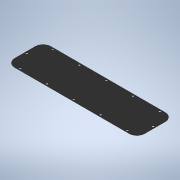
# Autodesk Inventor part: CAD_FPL_1060.000
Saved by Autodesk Inventor 2021 (Build 250183000, 183)
## iProperties
Created: 2025-09-22
Part Number: CAD_FPL_1060.000
Material: Generic
Catalog Web Link: www.cadenas.de
Description: Gland plate AX-Compact enclosures
Vendor: RITTAL
Document SubType Name: Modeling
Designer: psAdmin
Manufacturer: RITTAL
Mass: 117.298 g
Surface Area: 1587.71 cm^2
Volume: 117.298 cm^3
Density: 1 g/cm^3
Appearance: PSOLRGB-175-175-175
Category: PARTsolutions
Company: RITTAL
Title: CAD_FPL_1060.000
Author: Cadenas PARTsolutions
Comments: Compact enclosures
PSOL_IDENT_0: {$CADENAS_DATA/23d-libs/rittal/schaltschranksys/ausbauteile_cad/flanschplatten/ae_2_0_sep_fpl.prj},1
PSOL_IDENT_1: 81 {VTYP=3D},{NB=CAD_FPL_1060.000},{LINA=CAD_FPL_1060.000},{NN=Gland plate AX},{DATE=28.04.2025 21:1
PSOL_IDENT_2: 0:23},{GEOMDATE=11.04.2025 07:45:17},{VERSION=},{LINEID=350},{WBVAR=},{WBNUMERIC=}  {NB=CAD_FPL_1060
PSOL_IDENT_3: .000},{LINA=CAD_FPL_1060.000},{KT=DUMMY},{BEST=CAD_FPL_1060.000},{DETAIL=1},{VERS=7},{D=534},{E=149}
PSOL_IDENT_4: ,{BEZ1=Neues Kompaktgehäuse},{BEZ2=Stahlblech},{BEZ3=eintürig},{TUER=1},{B=600},{H=600},{T=210},{F=5
PSOL_IDENT_5: 50},{G=575},{B1=600},{B3=560.000},{B4=470.000},{B5=498.000},{BB5=0.000},{H1=600},{H3=560.000},{H4=85
PSOL_IDENT_6: .000},{H5=113.000},{HH5=4.000},{T5=93.500},{R1=31.000},{R2=8.000},{T1=210},{F1=550},{G1=575},{ST=MIN
PSOL_IDENT_7: },{VERS3=0},{CNSECLASS51=27-18-01-02},{CNSECLASS70=27-18-01-01},{CNSECLASS80=27-18-01-01},{CNSETIM40=
PSOL_IDENT_8: EC000261},{S=1.50},{W=600.000},{W1=556.000},{W2=500.000},{HH=600.000},{HH1=556.000},{HH2=550.000},{H
PSOL_IDENT_9: H3=475.000},{D1=205.100},{VERS1=1}
NB: CAD_FPL_1060.000
NN: Gland plate AX
NT: Compact enclosures
NBSYN: $BEST.
LINA: CAD_FPL_1060.000
CATALOG: Rittal
BEST: CAD_FPL_1060.000
D: 534
E: 149
SUPPLIER: RITTAL
ARTICLENO: CAD_FPL_1060.000
BOMINFO: CAD_FPL_1060.000
CREATOR: CADENAS GmbH
Autodesk Inventor part; units mm, degrees
(part 1 of 3)
sketch "Sketch_7" plane through (0, 0, 0) normal (0, 1, 0) x (1, 0, 0)
  arc A0 (-267, -42.5) -> (-235, -74.5) centre (-235, -42.5) ccw
  line L0 (-235, -74.5) -> (235, -74.5)
  arc A1 (235, -74.5) -> (267, -42.5) centre (235, -42.5) ccw
  line L1 (267, -42.5) -> (267, 42.5)
  arc A2 (267, 42.5) -> (235, 74.5) centre (235, 42.5) ccw
  line L2 (235, 74.5) -> (-235, 74.5)
  arc A3 (-235, 74.5) -> (-267, 42.5) centre (-235, 42.5) ccw
  line L3 (-267, 42.5) -> (-267, -42.5)
  circle A4 centre (259, 0) radius 3.6
  circle A5 centre (220, -66.5) radius 3.6
  circle A6 centre (220, 66.5) radius 3.6
  circle A7 centre (110, -66.5) radius 3.6
  circle A8 centre (110, 66.5) radius 3.6
  circle A9 centre (0, -66.5) radius 3.6
  circle A10 centre (0, 66.5) radius 3.6
  circle A11 centre (-110, -66.5) radius 3.6
  circle A12 centre (-110, 66.5) radius 3.6
  circle A13 centre (-220, -66.5) radius 3.6
  circle A14 centre (-220, 66.5) radius 3.6
  circle A15 centre (-259, 0) radius 3.6
  constraints: 16 centre point, 8 end point, 8 point on circle
extrude "Extrusion1" add sketch "Sketch_7" along normal blind 1.5
ref_plane "FP_XY" through (0, 0, 0) normal (0, -1, 0) x (1, 0, 0)
ref_plane "FP_YZ" through (0, 0, 0) normal (1, 0, 0) x (0, 0, 1)
ref_plane "FP_ZX" through (0, 0, 0) normal (0, 0, 1) x (0, -1, 0)
ref_plane "to_Bolt_1_XY" through (-300, 0, -300) normal (0, 1, 0) x (1, 0, 0)
ref_plane "to_Bolt_1_YZ" through (-300, 0, -300) normal (1, 0, 0) x (0, 0, -1)
ref_plane "to_Bolt_1_ZX" through (-300, 0, -300) normal (0, 0, -1) x (0, 1, 0)
ref_plane "to_Bolt_1_1_XY" through (-300, 0, -300) normal (0, 1, 0) x (1, 0, 0)
ref_plane "to_Bolt_1_1_YZ" through (-300, 0, -300) normal (1, 0, 0) x (0, 0, -1)
ref_plane "to_Bolt_1_1_ZX" through (-300, 0, -300) normal (0, 0, -1) x (0, 1, 0)
ref_plane "to_Bolt_1_10_XY" through (-274.1627, 0, -300) normal (0, 1, 0) x (1, 0, 0)
ref_plane "to_Bolt_1_10_YZ" through (-274.1627, 0, -300) normal (1, 0, 0) x (0, 0, -1)
ref_plane "to_Bolt_1_10_ZX" through (-274.1627, 0, -300) normal (0, 0, -1) x (0, 1, 0)
ref_plane "to_Bolt_1_100_XY" through (-15.7895, 0, -300) normal (0, 1, 0) x (1, 0, 0)
ref_plane "to_Bolt_1_100_YZ" through (-15.7895, 0, -300) normal (1, 0, 0) x (0, 0, -1)
ref_plane "to_Bolt_1_100_ZX" through (-15.7895, 0, -300) normal (0, 0, -1) x (0, 1, 0)
ref_plane "to_Bolt_1_101_XY" through (-12.9187, 0, -300) normal (0, 1, 0) x (1, 0, 0)
ref_plane "to_Bolt_1_101_YZ" through (-12.9187, 0, -300) normal (1, 0, 0) x (0, 0, -1)
ref_plane "to_Bolt_1_101_ZX" through (-12.9187, 0, -300) normal (0, 0, -1) x (0, 1, 0)
ref_plane "to_Bolt_1_102_XY" through (-10.0478, 0, -300) normal (0, 1, 0) x (1, 0, 0)
ref_plane "to_Bolt_1_102_YZ" through (-10.0478, 0, -300) normal (1, 0, 0) x (0, 0, -1)
ref_plane "to_Bolt_1_102_ZX" through (-10.0478, 0, -300) normal (0, 0, -1) x (0, 1, 0)
ref_plane "to_Bolt_1_103_XY" through (-7.177, 0, -300) normal (0, 1, 0) x (1, 0, 0)
ref_plane "to_Bolt_1_103_YZ" through (-7.177, 0, -300) normal (1, 0, 0) x (0, 0, -1)
ref_plane "to_Bolt_1_103_ZX" through (-7.177, 0, -300) normal (0, 0, -1) x (0, 1, 0)
ref_plane "to_Bolt_1_104_XY" through (-4.3062, 0, -300) normal (0, 1, 0) x (1, 0, 0)
ref_plane "to_Bolt_1_104_YZ" through (-4.3062, 0, -300) normal (1, 0, 0) x (0, 0, -1)
ref_plane "to_Bolt_1_104_ZX" through (-4.3062, 0, -300) normal (0, 0, -1) x (0, 1, 0)
ref_plane "to_Bolt_1_105_XY" through (-1.4354, 0, -300) normal (0, 1, 0) x (1, 0, 0)
ref_plane "to_Bolt_1_105_YZ" through (-1.4354, 0, -300) normal (1, 0, 0) x (0, 0, -1)
ref_plane "to_Bolt_1_105_ZX" through (-1.4354, 0, -300) normal (0, 0, -1) x (0, 1, 0)
ref_plane "to_Bolt_1_106_XY" through (1.4354, 0, -300) normal (0, 1, 0) x (1, 0, 0)
ref_plane "to_Bolt_1_106_YZ" through (1.4354, 0, -300) normal (1, 0, 0) x (0, 0, -1)
ref_plane "to_Bolt_1_106_ZX" through (1.4354, 0, -300) normal (0, 0, -1) x (0, 1, 0)
ref_plane "to_Bolt_1_107_XY" through (4.3062, 0, -300) normal (0, 1, 0) x (1, 0, 0)
ref_plane "to_Bolt_1_107_YZ" through (4.3062, 0, -300) normal (1, 0, 0) x (0, 0, -1)
ref_plane "to_Bolt_1_107_ZX" through (4.3062, 0, -300) normal (0, 0, -1) x (0, 1, 0)
ref_plane "to_Bolt_1_108_XY" through (7.177, 0, -300) normal (0, 1, 0) x (1, 0, 0)
ref_plane "to_Bolt_1_108_YZ" through (7.177, 0, -300) normal (1, 0, 0) x (0, 0, -1)
ref_plane "to_Bolt_1_108_ZX" through (7.177, 0, -300) normal (0, 0, -1) x (0, 1, 0)
ref_plane "to_Bolt_1_109_XY" through (10.0478, 0, -300) normal (0, 1, 0) x (1, 0, 0)
ref_plane "to_Bolt_1_109_YZ" through (10.0478, 0, -300) normal (1, 0, 0) x (0, 0, -1)
ref_plane "to_Bolt_1_109_ZX" through (10.0478, 0, -300) normal (0, 0, -1) x (0, 1, 0)
ref_plane "to_Bolt_1_11_XY" through (-271.2919, 0, -300) normal (0, 1, 0) x (1, 0, 0)
ref_plane "to_Bolt_1_11_YZ" through (-271.2919, 0, -300) normal (1, 0, 0) x (0, 0, -1)
ref_plane "to_Bolt_1_11_ZX" through (-271.2919, 0, -300) normal (0, 0, -1) x (0, 1, 0)
ref_plane "to_Bolt_1_110_XY" through (12.9187, 0, -300) normal (0, 1, 0) x (1, 0, 0)
ref_plane "to_Bolt_1_110_YZ" through (12.9187, 0, -300) normal (1, 0, 0) x (0, 0, -1)
ref_plane "to_Bolt_1_110_ZX" through (12.9187, 0, -300) normal (0, 0, -1) x (0, 1, 0)
ref_plane "to_Bolt_1_111_XY" through (15.7895, 0, -300) normal (0, 1, 0) x (1, 0, 0)
ref_plane "to_Bolt_1_111_YZ" through (15.7895, 0, -300) normal (1, 0, 0) x (0, 0, -1)
ref_plane "to_Bolt_1_111_ZX" through (15.7895, 0, -300) normal (0, 0, -1) x (0, 1, 0)
ref_plane "to_Bolt_1_112_XY" through (18.6603, 0, -300) normal (0, 1, 0) x (1, 0, 0)
ref_plane "to_Bolt_1_112_YZ" through (18.6603, 0, -300) normal (1, 0, 0) x (0, 0, -1)
ref_plane "to_Bolt_1_112_ZX" through (18.6603, 0, -300) normal (0, 0, -1) x (0, 1, 0)
ref_plane "to_Bolt_1_113_XY" through (21.5311, 0, -300) normal (0, 1, 0) x (1, 0, 0)
ref_plane "to_Bolt_1_113_YZ" through (21.5311, 0, -300) normal (1, 0, 0) x (0, 0, -1)
ref_plane "to_Bolt_1_113_ZX" through (21.5311, 0, -300) normal (0, 0, -1) x (0, 1, 0)
ref_plane "to_Bolt_1_114_XY" through (24.4019, 0, -300) normal (0, 1, 0) x (1, 0, 0)
ref_plane "to_Bolt_1_114_YZ" through (24.4019, 0, -300) normal (1, 0, 0) x (0, 0, -1)
ref_plane "to_Bolt_1_114_ZX" through (24.4019, 0, -300) normal (0, 0, -1) x (0, 1, 0)
ref_plane "to_Bolt_1_115_XY" through (27.2727, 0, -300) normal (0, 1, 0) x (1, 0, 0)
ref_plane "to_Bolt_1_115_YZ" through (27.2727, 0, -300) normal (1, 0, 0) x (0, 0, -1)
ref_plane "to_Bolt_1_115_ZX" through (27.2727, 0, -300) normal (0, 0, -1) x (0, 1, 0)
ref_plane "to_Bolt_1_116_XY" through (30.1435, 0, -300) normal (0, 1, 0) x (1, 0, 0)
ref_plane "to_Bolt_1_116_YZ" through (30.1435, 0, -300) normal (1, 0, 0) x (0, 0, -1)
ref_plane "to_Bolt_1_116_ZX" through (30.1435, 0, -300) normal (0, 0, -1) x (0, 1, 0)
ref_plane "to_Bolt_1_117_XY" through (33.0144, 0, -300) normal (0, 1, 0) x (1, 0, 0)
ref_plane "to_Bolt_1_117_YZ" through (33.0144, 0, -300) normal (1, 0, 0) x (0, 0, -1)
ref_plane "to_Bolt_1_117_ZX" through (33.0144, 0, -300) normal (0, 0, -1) x (0, 1, 0)
ref_plane "to_Bolt_1_118_XY" through (35.8852, 0, -300) normal (0, 1, 0) x (1, 0, 0)
ref_plane "to_Bolt_1_118_YZ" through (35.8852, 0, -300) normal (1, 0, 0) x (0, 0, -1)
ref_plane "to_Bolt_1_118_ZX" through (35.8852, 0, -300) normal (0, 0, -1) x (0, 1, 0)
ref_plane "to_Bolt_1_119_XY" through (38.756, 0, -300) normal (0, 1, 0) x (1, 0, 0)
ref_plane "to_Bolt_1_119_YZ" through (38.756, 0, -300) normal (1, 0, 0) x (0, 0, -1)
ref_plane "to_Bolt_1_119_ZX" through (38.756, 0, -300) normal (0, 0, -1) x (0, 1, 0)
ref_plane "to_Bolt_1_12_XY" through (-268.4211, 0, -300) normal (0, 1, 0) x (1, 0, 0)
ref_plane "to_Bolt_1_12_YZ" through (-268.4211, 0, -300) normal (1, 0, 0) x (0, 0, -1)
ref_plane "to_Bolt_1_12_ZX" through (-268.4211, 0, -300) normal (0, 0, -1) x (0, 1, 0)
ref_plane "to_Bolt_1_120_XY" through (41.6268, 0, -300) normal (0, 1, 0) x (1, 0, 0)
ref_plane "to_Bolt_1_120_YZ" through (41.6268, 0, -300) normal (1, 0, 0) x (0, 0, -1)
ref_plane "to_Bolt_1_120_ZX" through (41.6268, 0, -300) normal (0, 0, -1) x (0, 1, 0)
ref_plane "to_Bolt_1_121_XY" through (44.4976, 0, -300) normal (0, 1, 0) x (1, 0, 0)
ref_plane "to_Bolt_1_121_YZ" through (44.4976, 0, -300) normal (1, 0, 0) x (0, 0, -1)
ref_plane "to_Bolt_1_121_ZX" through (44.4976, 0, -300) normal (0, 0, -1) x (0, 1, 0)
ref_plane "to_Bolt_1_122_XY" through (47.3684, 0, -300) normal (0, 1, 0) x (1, 0, 0)
ref_plane "to_Bolt_1_122_YZ" through (47.3684, 0, -300) normal (1, 0, 0) x (0, 0, -1)
ref_plane "to_Bolt_1_122_ZX" through (47.3684, 0, -300) normal (0, 0, -1) x (0, 1, 0)
ref_plane "to_Bolt_1_123_XY" through (50.2392, 0, -300) normal (0, 1, 0) x (1, 0, 0)
ref_plane "to_Bolt_1_123_YZ" through (50.2392, 0, -300) normal (1, 0, 0) x (0, 0, -1)
ref_plane "to_Bolt_1_123_ZX" through (50.2392, 0, -300) normal (0, 0, -1) x (0, 1, 0)
ref_plane "to_Bolt_1_124_XY" through (53.11, 0, -300) normal (0, 1, 0) x (1, 0, 0)
ref_plane "to_Bolt_1_124_YZ" through (53.11, 0, -300) normal (1, 0, 0) x (0, 0, -1)
ref_plane "to_Bolt_1_124_ZX" through (53.11, 0, -300) normal (0, 0, -1) x (0, 1, 0)
ref_plane "to_Bolt_1_125_XY" through (55.9809, 0, -300) normal (0, 1, 0) x (1, 0, 0)
ref_plane "to_Bolt_1_125_YZ" through (55.9809, 0, -300) normal (1, 0, 0) x (0, 0, -1)
ref_plane "to_Bolt_1_125_ZX" through (55.9809, 0, -300) normal (0, 0, -1) x (0, 1, 0)
ref_plane "to_Bolt_1_126_XY" through (58.8517, 0, -300) normal (0, 1, 0) x (1, 0, 0)
ref_plane "to_Bolt_1_126_YZ" through (58.8517, 0, -300) normal (1, 0, 0) x (0, 0, -1)
ref_plane "to_Bolt_1_126_ZX" through (58.8517, 0, -300) normal (0, 0, -1) x (0, 1, 0)
ref_plane "to_Bolt_1_127_XY" through (61.7225, 0, -300) normal (0, 1, 0) x (1, 0, 0)
ref_plane "to_Bolt_1_127_YZ" through (61.7225, 0, -300) normal (1, 0, 0) x (0, 0, -1)
ref_plane "to_Bolt_1_127_ZX" through (61.7225, 0, -300) normal (0, 0, -1) x (0, 1, 0)
ref_plane "to_Bolt_1_128_XY" through (64.5933, 0, -300) normal (0, 1, 0) x (1, 0, 0)
ref_plane "to_Bolt_1_128_YZ" through (64.5933, 0, -300) normal (1, 0, 0) x (0, 0, -1)
ref_plane "to_Bolt_1_128_ZX" through (64.5933, 0, -300) normal (0, 0, -1) x (0, 1, 0)
ref_plane "to_Bolt_1_129_XY" through (67.4641, 0, -300) normal (0, 1, 0) x (1, 0, 0)
ref_plane "to_Bolt_1_129_YZ" through (67.4641, 0, -300) normal (1, 0, 0) x (0, 0, -1)
ref_plane "to_Bolt_1_129_ZX" through (67.4641, 0, -300) normal (0, 0, -1) x (0, 1, 0)
ref_plane "to_Bolt_1_13_XY" through (-265.5502, 0, -300) normal (0, 1, 0) x (1, 0, 0)
ref_plane "to_Bolt_1_13_YZ" through (-265.5502, 0, -300) normal (1, 0, 0) x (0, 0, -1)
ref_plane "to_Bolt_1_13_ZX" through (-265.5502, 0, -300) normal (0, 0, -1) x (0, 1, 0)
ref_plane "to_Bolt_1_130_XY" through (70.3349, 0, -300) normal (0, 1, 0) x (1, 0, 0)
ref_plane "to_Bolt_1_130_YZ" through (70.3349, 0, -300) normal (1, 0, 0) x (0, 0, -1)
ref_plane "to_Bolt_1_130_ZX" through (70.3349, 0, -300) normal (0, 0, -1) x (0, 1, 0)
ref_plane "to_Bolt_1_131_XY" through (73.2057, 0, -300) normal (0, 1, 0) x (1, 0, 0)
ref_plane "to_Bolt_1_131_YZ" through (73.2057, 0, -300) normal (1, 0, 0) x (0, 0, -1)
ref_plane "to_Bolt_1_131_ZX" through (73.2057, 0, -300) normal (0, 0, -1) x (0, 1, 0)
ref_plane "to_Bolt_1_132_XY" through (76.0766, 0, -300) normal (0, 1, 0) x (1, 0, 0)
ref_plane "to_Bolt_1_132_YZ" through (76.0766, 0, -300) normal (1, 0, 0) x (0, 0, -1)
ref_plane "to_Bolt_1_132_ZX" through (76.0766, 0, -300) normal (0, 0, -1) x (0, 1, 0)
ref_plane "to_Bolt_1_133_XY" through (78.9474, 0, -300) normal (0, 1, 0) x (1, 0, 0)
ref_plane "to_Bolt_1_133_YZ" through (78.9474, 0, -300) normal (1, 0, 0) x (0, 0, -1)
ref_plane "to_Bolt_1_133_ZX" through (78.9474, 0, -300) normal (0, 0, -1) x (0, 1, 0)
ref_plane "to_Bolt_1_134_XY" through (81.8182, 0, -300) normal (0, 1, 0) x (1, 0, 0)
ref_plane "to_Bolt_1_134_YZ" through (81.8182, 0, -300) normal (1, 0, 0) x (0, 0, -1)
ref_plane "to_Bolt_1_134_ZX" through (81.8182, 0, -300) normal (0, 0, -1) x (0, 1, 0)
ref_plane "to_Bolt_1_135_XY" through (84.689, 0, -300) normal (0, 1, 0) x (1, 0, 0)
ref_plane "to_Bolt_1_135_YZ" through (84.689, 0, -300) normal (1, 0, 0) x (0, 0, -1)
ref_plane "to_Bolt_1_135_ZX" through (84.689, 0, -300) normal (0, 0, -1) x (0, 1, 0)
ref_plane "to_Bolt_1_136_XY" through (87.5598, 0, -300) normal (0, 1, 0) x (1, 0, 0)
ref_plane "to_Bolt_1_136_YZ" through (87.5598, 0, -300) normal (1, 0, 0) x (0, 0, -1)
ref_plane "to_Bolt_1_136_ZX" through (87.5598, 0, -300) normal (0, 0, -1) x (0, 1, 0)
ref_plane "to_Bolt_1_137_XY" through (90.4306, 0, -300) normal (0, 1, 0) x (1, 0, 0)
ref_plane "to_Bolt_1_137_YZ" through (90.4306, 0, -300) normal (1, 0, 0) x (0, 0, -1)
ref_plane "to_Bolt_1_137_ZX" through (90.4306, 0, -300) normal (0, 0, -1) x (0, 1, 0)
ref_plane "to_Bolt_1_138_XY" through (93.3014, 0, -300) normal (0, 1, 0) x (1, 0, 0)
ref_plane "to_Bolt_1_138_YZ" through (93.3014, 0, -300) normal (1, 0, 0) x (0, 0, -1)
ref_plane "to_Bolt_1_138_ZX" through (93.3014, 0, -300) normal (0, 0, -1) x (0, 1, 0)
ref_plane "to_Bolt_1_139_XY" through (96.1722, 0, -300) normal (0, 1, 0) x (1, 0, 0)
ref_plane "to_Bolt_1_139_YZ" through (96.1722, 0, -300) normal (1, 0, 0) x (0, 0, -1)
ref_plane "to_Bolt_1_139_ZX" through (96.1722, 0, -300) normal (0, 0, -1) x (0, 1, 0)
ref_plane "to_Bolt_1_14_XY" through (-262.6794, 0, -300) normal (0, 1, 0) x (1, 0, 0)
ref_plane "to_Bolt_1_14_YZ" through (-262.6794, 0, -300) normal (1, 0, 0) x (0, 0, -1)
ref_plane "to_Bolt_1_14_ZX" through (-262.6794, 0, -300) normal (0, 0, -1) x (0, 1, 0)
ref_plane "to_Bolt_1_140_XY" through (99.0431, 0, -300) normal (0, 1, 0) x (1, 0, 0)
ref_plane "to_Bolt_1_140_YZ" through (99.0431, 0, -300) normal (1, 0, 0) x (0, 0, -1)
ref_plane "to_Bolt_1_140_ZX" through (99.0431, 0, -300) normal (0, 0, -1) x (0, 1, 0)
ref_plane "to_Bolt_1_141_XY" through (101.9139, 0, -300) normal (0, 1, 0) x (1, 0, 0)
ref_plane "to_Bolt_1_141_YZ" through (101.9139, 0, -300) normal (1, 0, 0) x (0, 0, -1)
ref_plane "to_Bolt_1_141_ZX" through (101.9139, 0, -300) normal (0, 0, -1) x (0, 1, 0)
ref_plane "to_Bolt_1_142_XY" through (104.7847, 0, -300) normal (0, 1, 0) x (1, 0, 0)
ref_plane "to_Bolt_1_142_YZ" through (104.7847, 0, -300) normal (1, 0, 0) x (0, 0, -1)
ref_plane "to_Bolt_1_142_ZX" through (104.7847, 0, -300) normal (0, 0, -1) x (0, 1, 0)
ref_plane "to_Bolt_1_143_XY" through (107.6555, 0, -300) normal (0, 1, 0) x (1, 0, 0)
ref_plane "to_Bolt_1_143_YZ" through (107.6555, 0, -300) normal (1, 0, 0) x (0, 0, -1)
ref_plane "to_Bolt_1_143_ZX" through (107.6555, 0, -300) normal (0, 0, -1) x (0, 1, 0)
ref_plane "to_Bolt_1_144_XY" through (110.5263, 0, -300) normal (0, 1, 0) x (1, 0, 0)
ref_plane "to_Bolt_1_144_YZ" through (110.5263, 0, -300) normal (1, 0, 0) x (0, 0, -1)
ref_plane "to_Bolt_1_144_ZX" through (110.5263, 0, -300) normal (0, 0, -1) x (0, 1, 0)
ref_plane "to_Bolt_1_145_XY" through (113.3971, 0, -300) normal (0, 1, 0) x (1, 0, 0)
ref_plane "to_Bolt_1_145_YZ" through (113.3971, 0, -300) normal (1, 0, 0) x (0, 0, -1)
ref_plane "to_Bolt_1_145_ZX" through (113.3971, 0, -300) normal (0, 0, -1) x (0, 1, 0)
ref_plane "to_Bolt_1_146_XY" through (116.2679, 0, -300) normal (0, 1, 0) x (1, 0, 0)
ref_plane "to_Bolt_1_146_YZ" through (116.2679, 0, -300) normal (1, 0, 0) x (0, 0, -1)
ref_plane "to_Bolt_1_146_ZX" through (116.2679, 0, -300) normal (0, 0, -1) x (0, 1, 0)
ref_plane "to_Bolt_1_147_XY" through (119.1388, 0, -300) normal (0, 1, 0) x (1, 0, 0)
ref_plane "to_Bolt_1_147_YZ" through (119.1388, 0, -300) normal (1, 0, 0) x (0, 0, -1)
ref_plane "to_Bolt_1_147_ZX" through (119.1388, 0, -300) normal (0, 0, -1) x (0, 1, 0)
ref_plane "to_Bolt_1_148_XY" through (122.0096, 0, -300) normal (0, 1, 0) x (1, 0, 0)
ref_plane "to_Bolt_1_148_YZ" through (122.0096, 0, -300) normal (1, 0, 0) x (0, 0, -1)
ref_plane "to_Bolt_1_148_ZX" through (122.0096, 0, -300) normal (0, 0, -1) x (0, 1, 0)
ref_plane "to_Bolt_1_149_XY" through (124.8804, 0, -300) normal (0, 1, 0) x (1, 0, 0)
ref_plane "to_Bolt_1_149_YZ" through (124.8804, 0, -300) normal (1, 0, 0) x (0, 0, -1)
ref_plane "to_Bolt_1_149_ZX" through (124.8804, 0, -300) normal (0, 0, -1) x (0, 1, 0)
ref_plane "to_Bolt_1_15_XY" through (-259.8086, 0, -300) normal (0, 1, 0) x (1, 0, 0)
ref_plane "to_Bolt_1_15_YZ" through (-259.8086, 0, -300) normal (1, 0, 0) x (0, 0, -1)
ref_plane "to_Bolt_1_15_ZX" through (-259.8086, 0, -300) normal (0, 0, -1) x (0, 1, 0)
ref_plane "to_Bolt_1_150_XY" through (127.7512, 0, -300) normal (0, 1, 0) x (1, 0, 0)
ref_plane "to_Bolt_1_150_YZ" through (127.7512, 0, -300) normal (1, 0, 0) x (0, 0, -1)
ref_plane "to_Bolt_1_150_ZX" through (127.7512, 0, -300) normal (0, 0, -1) x (0, 1, 0)
ref_plane "to_Bolt_1_151_XY" through (130.622, 0, -300) normal (0, 1, 0) x (1, 0, 0)
ref_plane "to_Bolt_1_151_YZ" through (130.622, 0, -300) normal (1, 0, 0) x (0, 0, -1)
ref_plane "to_Bolt_1_151_ZX" through (130.622, 0, -300) normal (0, 0, -1) x (0, 1, 0)
ref_plane "to_Bolt_1_152_XY" through (133.4928, 0, -300) normal (0, 1, 0) x (1, 0, 0)
ref_plane "to_Bolt_1_152_YZ" through (133.4928, 0, -300) normal (1, 0, 0) x (0, 0, -1)
ref_plane "to_Bolt_1_152_ZX" through (133.4928, 0, -300) normal (0, 0, -1) x (0, 1, 0)
ref_plane "to_Bolt_1_153_XY" through (136.3636, 0, -300) normal (0, 1, 0) x (1, 0, 0)
ref_plane "to_Bolt_1_153_YZ" through (136.3636, 0, -300) normal (1, 0, 0) x (0, 0, -1)
ref_plane "to_Bolt_1_153_ZX" through (136.3636, 0, -300) normal (0, 0, -1) x (0, 1, 0)
ref_plane "to_Bolt_1_154_XY" through (139.2344, 0, -300) normal (0, 1, 0) x (1, 0, 0)
ref_plane "to_Bolt_1_154_YZ" through (139.2344, 0, -300) normal (1, 0, 0) x (0, 0, -1)
ref_plane "to_Bolt_1_154_ZX" through (139.2344, 0, -300) normal (0, 0, -1) x (0, 1, 0)
ref_plane "to_Bolt_1_155_XY" through (142.1053, 0, -300) normal (0, 1, 0) x (1, 0, 0)
ref_plane "to_Bolt_1_155_YZ" through (142.1053, 0, -300) normal (1, 0, 0) x (0, 0, -1)
ref_plane "to_Bolt_1_155_ZX" through (142.1053, 0, -300) normal (0, 0, -1) x (0, 1, 0)
ref_plane "to_Bolt_1_156_XY" through (144.9761, 0, -300) normal (0, 1, 0) x (1, 0, 0)
ref_plane "to_Bolt_1_156_YZ" through (144.9761, 0, -300) normal (1, 0, 0) x (0, 0, -1)
ref_plane "to_Bolt_1_156_ZX" through (144.9761, 0, -300) normal (0, 0, -1) x (0, 1, 0)
ref_plane "to_Bolt_1_157_XY" through (147.8469, 0, -300) normal (0, 1, 0) x (1, 0, 0)
ref_plane "to_Bolt_1_157_YZ" through (147.8469, 0, -300) normal (1, 0, 0) x (0, 0, -1)
ref_plane "to_Bolt_1_157_ZX" through (147.8469, 0, -300) normal (0, 0, -1) x (0, 1, 0)
ref_plane "to_Bolt_1_158_XY" through (150.7177, 0, -300) normal (0, 1, 0) x (1, 0, 0)
ref_plane "to_Bolt_1_158_YZ" through (150.7177, 0, -300) normal (1, 0, 0) x (0, 0, -1)
ref_plane "to_Bolt_1_158_ZX" through (150.7177, 0, -300) normal (0, 0, -1) x (0, 1, 0)
ref_plane "to_Bolt_1_159_XY" through (153.5885, 0, -300) normal (0, 1, 0) x (1, 0, 0)
ref_plane "to_Bolt_1_159_YZ" through (153.5885, 0, -300) normal (1, 0, 0) x (0, 0, -1)
ref_plane "to_Bolt_1_159_ZX" through (153.5885, 0, -300) normal (0, 0, -1) x (0, 1, 0)
ref_plane "to_Bolt_1_16_XY" through (-256.9378, 0, -300) normal (0, 1, 0) x (1, 0, 0)
ref_plane "to_Bolt_1_16_YZ" through (-256.9378, 0, -300) normal (1, 0, 0) x (0, 0, -1)
ref_plane "to_Bolt_1_16_ZX" through (-256.9378, 0, -300) normal (0, 0, -1) x (0, 1, 0)
ref_plane "to_Bolt_1_160_XY" through (156.4593, 0, -300) normal (0, 1, 0) x (1, 0, 0)
ref_plane "to_Bolt_1_160_YZ" through (156.4593, 0, -300) normal (1, 0, 0) x (0, 0, -1)
ref_plane "to_Bolt_1_160_ZX" through (156.4593, 0, -300) normal (0, 0, -1) x (0, 1, 0)
ref_plane "to_Bolt_1_161_XY" through (159.3301, 0, -300) normal (0, 1, 0) x (1, 0, 0)
ref_plane "to_Bolt_1_161_YZ" through (159.3301, 0, -300) normal (1, 0, 0) x (0, 0, -1)
ref_plane "to_Bolt_1_161_ZX" through (159.3301, 0, -300) normal (0, 0, -1) x (0, 1, 0)
ref_plane "to_Bolt_1_162_XY" through (162.201, 0, -300) normal (0, 1, 0) x (1, 0, 0)
ref_plane "to_Bolt_1_162_YZ" through (162.201, 0, -300) normal (1, 0, 0) x (0, 0, -1)
ref_plane "to_Bolt_1_162_ZX" through (162.201, 0, -300) normal (0, 0, -1) x (0, 1, 0)
ref_plane "to_Bolt_1_163_XY" through (165.0718, 0, -300) normal (0, 1, 0) x (1, 0, 0)
ref_plane "to_Bolt_1_163_YZ" through (165.0718, 0, -300) normal (1, 0, 0) x (0, 0, -1)
ref_plane "to_Bolt_1_163_ZX" through (165.0718, 0, -300) normal (0, 0, -1) x (0, 1, 0)
ref_plane "to_Bolt_1_164_XY" through (167.9426, 0, -300) normal (0, 1, 0) x (1, 0, 0)
ref_plane "to_Bolt_1_164_YZ" through (167.9426, 0, -300) normal (1, 0, 0) x (0, 0, -1)
ref_plane "to_Bolt_1_164_ZX" through (167.9426, 0, -300) normal (0, 0, -1) x (0, 1, 0)
ref_plane "to_Bolt_1_165_XY" through (170.8134, 0, -300) normal (0, 1, 0) x (1, 0, 0)
ref_plane "to_Bolt_1_165_YZ" through (170.8134, 0, -300) normal (1, 0, 0) x (0, 0, -1)
ref_plane "to_Bolt_1_165_ZX" through (170.8134, 0, -300) normal (0, 0, -1) x (0, 1, 0)
ref_plane "to_Bolt_1_166_XY" through (173.6842, 0, -300) normal (0, 1, 0) x (1, 0, 0)
ref_plane "to_Bolt_1_166_YZ" through (173.6842, 0, -300) normal (1, 0, 0) x (0, 0, -1)
ref_plane "to_Bolt_1_166_ZX" through (173.6842, 0, -300) normal (0, 0, -1) x (0, 1, 0)
ref_plane "to_Bolt_1_167_XY" through (176.555, 0, -300) normal (0, 1, 0) x (1, 0, 0)
ref_plane "to_Bolt_1_167_YZ" through (176.555, 0, -300) normal (1, 0, 0) x (0, 0, -1)
ref_plane "to_Bolt_1_167_ZX" through (176.555, 0, -300) normal (0, 0, -1) x (0, 1, 0)
ref_plane "to_Bolt_1_168_XY" through (179.4258, 0, -300) normal (0, 1, 0) x (1, 0, 0)
ref_plane "to_Bolt_1_168_YZ" through (179.4258, 0, -300) normal (1, 0, 0) x (0, 0, -1)
ref_plane "to_Bolt_1_168_ZX" through (179.4258, 0, -300) normal (0, 0, -1) x (0, 1, 0)
ref_plane "to_Bolt_1_169_XY" through (182.2967, 0, -300) normal (0, 1, 0) x (1, 0, 0)
ref_plane "to_Bolt_1_169_YZ" through (182.2967, 0, -300) normal (1, 0, 0) x (0, 0, -1)
ref_plane "to_Bolt_1_169_ZX" through (182.2967, 0, -300) normal (0, 0, -1) x (0, 1, 0)
ref_plane "to_Bolt_1_17_XY" through (-254.067, 0, -300) normal (0, 1, 0) x (1, 0, 0)
ref_plane "to_Bolt_1_17_YZ" through (-254.067, 0, -300) normal (1, 0, 0) x (0, 0, -1)
ref_plane "to_Bolt_1_17_ZX" through (-254.067, 0, -300) normal (0, 0, -1) x (0, 1, 0)
ref_plane "to_Bolt_1_170_XY" through (185.1675, 0, -300) normal (0, 1, 0) x (1, 0, 0)
ref_plane "to_Bolt_1_170_YZ" through (185.1675, 0, -300) normal (1, 0, 0) x (0, 0, -1)
ref_plane "to_Bolt_1_170_ZX" through (185.1675, 0, -300) normal (0, 0, -1) x (0, 1, 0)
ref_plane "to_Bolt_1_171_XY" through (188.0383, 0, -300) normal (0, 1, 0) x (1, 0, 0)
ref_plane "to_Bolt_1_171_YZ" through (188.0383, 0, -300) normal (1, 0, 0) x (0, 0, -1)
ref_plane "to_Bolt_1_171_ZX" through (188.0383, 0, -300) normal (0, 0, -1) x (0, 1, 0)
ref_plane "to_Bolt_1_172_XY" through (190.9091, 0, -300) normal (0, 1, 0) x (1, 0, 0)
ref_plane "to_Bolt_1_172_YZ" through (190.9091, 0, -300) normal (1, 0, 0) x (0, 0, -1)
ref_plane "to_Bolt_1_172_ZX" through (190.9091, 0, -300) normal (0, 0, -1) x (0, 1, 0)
ref_plane "to_Bolt_1_173_XY" through (193.7799, 0, -300) normal (0, 1, 0) x (1, 0, 0)
ref_plane "to_Bolt_1_173_YZ" through (193.7799, 0, -300) normal (1, 0, 0) x (0, 0, -1)
ref_plane "to_Bolt_1_173_ZX" through (193.7799, 0, -300) normal (0, 0, -1) x (0, 1, 0)
ref_plane "to_Bolt_1_174_XY" through (196.6507, 0, -300) normal (0, 1, 0) x (1, 0, 0)
ref_plane "to_Bolt_1_174_YZ" through (196.6507, 0, -300) normal (1, 0, 0) x (0, 0, -1)
ref_plane "to_Bolt_1_174_ZX" through (196.6507, 0, -300) normal (0, 0, -1) x (0, 1, 0)
ref_plane "to_Bolt_1_175_XY" through (199.5215, 0, -300) normal (0, 1, 0) x (1, 0, 0)
ref_plane "to_Bolt_1_175_YZ" through (199.5215, 0, -300) normal (1, 0, 0) x (0, 0, -1)
ref_plane "to_Bolt_1_175_ZX" through (199.5215, 0, -300) normal (0, 0, -1) x (0, 1, 0)
ref_plane "to_Bolt_1_176_XY" through (202.3923, 0, -300) normal (0, 1, 0) x (1, 0, 0)
ref_plane "to_Bolt_1_176_YZ" through (202.3923, 0, -300) normal (1, 0, 0) x (0, 0, -1)
ref_plane "to_Bolt_1_176_ZX" through (202.3923, 0, -300) normal (0, 0, -1) x (0, 1, 0)
ref_plane "to_Bolt_1_177_XY" through (205.2632, 0, -300) normal (0, 1, 0) x (1, 0, 0)
ref_plane "to_Bolt_1_177_YZ" through (205.2632, 0, -300) normal (1, 0, 0) x (0, 0, -1)
ref_plane "to_Bolt_1_177_ZX" through (205.2632, 0, -300) normal (0, 0, -1) x (0, 1, 0)
ref_plane "to_Bolt_1_178_XY" through (208.134, 0, -300) normal (0, 1, 0) x (1, 0, 0)
ref_plane "to_Bolt_1_178_YZ" through (208.134, 0, -300) normal (1, 0, 0) x (0, 0, -1)
ref_plane "to_Bolt_1_178_ZX" through (208.134, 0, -300) normal (0, 0, -1) x (0, 1, 0)
ref_plane "to_Bolt_1_179_XY" through (211.0048, 0, -300) normal (0, 1, 0) x (1, 0, 0)
ref_plane "to_Bolt_1_179_YZ" through (211.0048, 0, -300) normal (1, 0, 0) x (0, 0, -1)
ref_plane "to_Bolt_1_179_ZX" through (211.0048, 0, -300) normal (0, 0, -1) x (0, 1, 0)
ref_plane "to_Bolt_1_18_XY" through (-251.1962, 0, -300) normal (0, 1, 0) x (1, 0, 0)
ref_plane "to_Bolt_1_18_YZ" through (-251.1962, 0, -300) normal (1, 0, 0) x (0, 0, -1)
ref_plane "to_Bolt_1_18_ZX" through (-251.1962, 0, -300) normal (0, 0, -1) x (0, 1, 0)
ref_plane "to_Bolt_1_180_XY" through (213.8756, 0, -300) normal (0, 1, 0) x (1, 0, 0)
ref_plane "to_Bolt_1_180_YZ" through (213.8756, 0, -300) normal (1, 0, 0) x (0, 0, -1)
ref_plane "to_Bolt_1_180_ZX" through (213.8756, 0, -300) normal (0, 0, -1) x (0, 1, 0)
ref_plane "to_Bolt_1_181_XY" through (216.7464, 0, -300) normal (0, 1, 0) x (1, 0, 0)
ref_plane "to_Bolt_1_181_YZ" through (216.7464, 0, -300) normal (1, 0, 0) x (0, 0, -1)
ref_plane "to_Bolt_1_181_ZX" through (216.7464, 0, -300) normal (0, 0, -1) x (0, 1, 0)
ref_plane "to_Bolt_1_182_XY" through (219.6172, 0, -300) normal (0, 1, 0) x (1, 0, 0)
ref_plane "to_Bolt_1_182_YZ" through (219.6172, 0, -300) normal (1, 0, 0) x (0, 0, -1)
ref_plane "to_Bolt_1_182_ZX" through (219.6172, 0, -300) normal (0, 0, -1) x (0, 1, 0)
ref_plane "to_Bolt_1_183_XY" through (222.488, 0, -300) normal (0, 1, 0) x (1, 0, 0)
ref_plane "to_Bolt_1_183_YZ" through (222.488, 0, -300) normal (1, 0, 0) x (0, 0, -1)
ref_plane "to_Bolt_1_183_ZX" through (222.488, 0, -300) normal (0, 0, -1) x (0, 1, 0)
ref_plane "to_Bolt_1_184_XY" through (225.3589, 0, -300) normal (0, 1, 0) x (1, 0, 0)
ref_plane "to_Bolt_1_184_YZ" through (225.3589, 0, -300) normal (1, 0, 0) x (0, 0, -1)
ref_plane "to_Bolt_1_184_ZX" through (225.3589, 0, -300) normal (0, 0, -1) x (0, 1, 0)
ref_plane "to_Bolt_1_185_XY" through (228.2297, 0, -300) normal (0, 1, 0) x (1, 0, 0)
ref_plane "to_Bolt_1_185_YZ" through (228.2297, 0, -300) normal (1, 0, 0) x (0, 0, -1)
ref_plane "to_Bolt_1_185_ZX" through (228.2297, 0, -300) normal (0, 0, -1) x (0, 1, 0)
ref_plane "to_Bolt_1_186_XY" through (231.1005, 0, -300) normal (0, 1, 0) x (1, 0, 0)
ref_plane "to_Bolt_1_186_YZ" through (231.1005, 0, -300) normal (1, 0, 0) x (0, 0, -1)
ref_plane "to_Bolt_1_186_ZX" through (231.1005, 0, -300) normal (0, 0, -1) x (0, 1, 0)
ref_plane "to_Bolt_1_187_XY" through (233.9713, 0, -300) normal (0, 1, 0) x (1, 0, 0)
ref_plane "to_Bolt_1_187_YZ" through (233.9713, 0, -300) normal (1, 0, 0) x (0, 0, -1)
ref_plane "to_Bolt_1_187_ZX" through (233.9713, 0, -300) normal (0, 0, -1) x (0, 1, 0)
ref_plane "to_Bolt_1_188_XY" through (236.8421, 0, -300) normal (0, 1, 0) x (1, 0, 0)
ref_plane "to_Bolt_1_188_YZ" through (236.8421, 0, -300) normal (1, 0, 0) x (0, 0, -1)
ref_plane "to_Bolt_1_188_ZX" through (236.8421, 0, -300) normal (0, 0, -1) x (0, 1, 0)
ref_plane "to_Bolt_1_189_XY" through (239.7129, 0, -300) normal (0, 1, 0) x (1, 0, 0)
ref_plane "to_Bolt_1_189_YZ" through (239.7129, 0, -300) normal (1, 0, 0) x (0, 0, -1)
ref_plane "to_Bolt_1_189_ZX" through (239.7129, 0, -300) normal (0, 0, -1) x (0, 1, 0)
ref_plane "to_Bolt_1_19_XY" through (-248.3254, 0, -300) normal (0, 1, 0) x (1, 0, 0)
ref_plane "to_Bolt_1_19_YZ" through (-248.3254, 0, -300) normal (1, 0, 0) x (0, 0, -1)
ref_plane "to_Bolt_1_19_ZX" through (-248.3254, 0, -300) normal (0, 0, -1) x (0, 1, 0)
ref_plane "to_Bolt_1_190_XY" through (242.5837, 0, -300) normal (0, 1, 0) x (1, 0, 0)
ref_plane "to_Bolt_1_190_YZ" through (242.5837, 0, -300) normal (1, 0, 0) x (0, 0, -1)
ref_plane "to_Bolt_1_190_ZX" through (242.5837, 0, -300) normal (0, 0, -1) x (0, 1, 0)
ref_plane "to_Bolt_1_191_XY" through (245.4545, 0, -300) normal (0, 1, 0) x (1, 0, 0)
ref_plane "to_Bolt_1_191_YZ" through (245.4545, 0, -300) normal (1, 0, 0) x (0, 0, -1)
ref_plane "to_Bolt_1_191_ZX" through (245.4545, 0, -300) normal (0, 0, -1) x (0, 1, 0)
ref_plane "to_Bolt_1_192_XY" through (248.3254, 0, -300) normal (0, 1, 0) x (1, 0, 0)
ref_plane "to_Bolt_1_192_YZ" through (248.3254, 0, -300) normal (1, 0, 0) x (0, 0, -1)
ref_plane "to_Bolt_1_192_ZX" through (248.3254, 0, -300) normal (0, 0, -1) x (0, 1, 0)
ref_plane "to_Bolt_1_193_XY" through (251.1962, 0, -300) normal (0, 1, 0) x (1, 0, 0)
ref_plane "to_Bolt_1_193_YZ" through (251.1962, 0, -300) normal (1, 0, 0) x (0, 0, -1)
ref_plane "to_Bolt_1_193_ZX" through (251.1962, 0, -300) normal (0, 0, -1) x (0, 1, 0)
ref_plane "to_Bolt_1_194_XY" through (254.067, 0, -300) normal (0, 1, 0) x (1, 0, 0)
ref_plane "to_Bolt_1_194_YZ" through (254.067, 0, -300) normal (1, 0, 0) x (0, 0, -1)
ref_plane "to_Bolt_1_194_ZX" through (254.067, 0, -300) normal (0, 0, -1) x (0, 1, 0)
ref_plane "to_Bolt_1_195_XY" through (256.9378, 0, -300) normal (0, 1, 0) x (1, 0, 0)
ref_plane "to_Bolt_1_195_YZ" through (256.9378, 0, -300) normal (1, 0, 0) x (0, 0, -1)
ref_plane "to_Bolt_1_195_ZX" through (256.9378, 0, -300) normal (0, 0, -1) x (0, 1, 0)
ref_plane "to_Bolt_1_196_XY" through (259.8086, 0, -300) normal (0, 1, 0) x (1, 0, 0)
ref_plane "to_Bolt_1_196_YZ" through (259.8086, 0, -300) normal (1, 0, 0) x (0, 0, -1)
ref_plane "to_Bolt_1_196_ZX" through (259.8086, 0, -300) normal (0, 0, -1) x (0, 1, 0)
ref_plane "to_Bolt_1_197_XY" through (262.6794, 0, -300) normal (0, 1, 0) x (1, 0, 0)
ref_plane "to_Bolt_1_197_YZ" through (262.6794, 0, -300) normal (1, 0, 0) x (0, 0, -1)
ref_plane "to_Bolt_1_197_ZX" through (262.6794, 0, -300) normal (0, 0, -1) x (0, 1, 0)
ref_plane "to_Bolt_1_198_XY" through (265.5502, 0, -300) normal (0, 1, 0) x (1, 0, 0)
ref_plane "to_Bolt_1_198_YZ" through (265.5502, 0, -300) normal (1, 0, 0) x (0, 0, -1)
ref_plane "to_Bolt_1_198_ZX" through (265.5502, 0, -300) normal (0, 0, -1) x (0, 1, 0)
ref_plane "to_Bolt_1_199_XY" through (268.4211, 0, -300) normal (0, 1, 0) x (1, 0, 0)
ref_plane "to_Bolt_1_199_YZ" through (268.4211, 0, -300) normal (1, 0, 0) x (0, 0, -1)
ref_plane "to_Bolt_1_199_ZX" through (268.4211, 0, -300) normal (0, 0, -1) x (0, 1, 0)
ref_plane "to_Bolt_1_2_XY" through (-297.1292, 0, -300) normal (0, 1, 0) x (1, 0, 0)
ref_plane "to_Bolt_1_2_YZ" through (-297.1292, 0, -300) normal (1, 0, 0) x (0, 0, -1)
ref_plane "to_Bolt_1_2_ZX" through (-297.1292, 0, -300) normal (0, 0, -1) x (0, 1, 0)
ref_plane "to_Bolt_1_20_XY" through (-245.4545, 0, -300) normal (0, 1, 0) x (1, 0, 0)
ref_plane "to_Bolt_1_20_YZ" through (-245.4545, 0, -300) normal (1, 0, 0) x (0, 0, -1)
ref_plane "to_Bolt_1_20_ZX" through (-245.4545, 0, -300) normal (0, 0, -1) x (0, 1, 0)
ref_plane "to_Bolt_1_200_XY" through (271.2919, 0, -300) normal (0, 1, 0) x (1, 0, 0)
ref_plane "to_Bolt_1_200_YZ" through (271.2919, 0, -300) normal (1, 0, 0) x (0, 0, -1)
ref_plane "to_Bolt_1_200_ZX" through (271.2919, 0, -300) normal (0, 0, -1) x (0, 1, 0)
ref_plane "to_Bolt_1_201_XY" through (274.1627, 0, -300) normal (0, 1, 0) x (1, 0, 0)
ref_plane "to_Bolt_1_201_YZ" through (274.1627, 0, -300) normal (1, 0, 0) x (0, 0, -1)
ref_plane "to_Bolt_1_201_ZX" through (274.1627, 0, -300) normal (0, 0, -1) x (0, 1, 0)
ref_plane "to_Bolt_1_202_XY" through (277.0335, 0, -300) normal (0, 1, 0) x (1, 0, 0)
ref_plane "to_Bolt_1_202_YZ" through (277.0335, 0, -300) normal (1, 0, 0) x (0, 0, -1)
ref_plane "to_Bolt_1_202_ZX" through (277.0335, 0, -300) normal (0, 0, -1) x (0, 1, 0)
ref_plane "to_Bolt_1_203_XY" through (279.9043, 0, -300) normal (0, 1, 0) x (1, 0, 0)
ref_plane "to_Bolt_1_203_YZ" through (279.9043, 0, -300) normal (1, 0, 0) x (0, 0, -1)
ref_plane "to_Bolt_1_203_ZX" through (279.9043, 0, -300) normal (0, 0, -1) x (0, 1, 0)
ref_plane "to_Bolt_1_204_XY" through (282.7751, 0, -300) normal (0, 1, 0) x (1, 0, 0)
ref_plane "to_Bolt_1_204_YZ" through (282.7751, 0, -300) normal (1, 0, 0) x (0, 0, -1)
ref_plane "to_Bolt_1_204_ZX" through (282.7751, 0, -300) normal (0, 0, -1) x (0, 1, 0)
ref_plane "to_Bolt_1_205_XY" through (285.6459, 0, -300) normal (0, 1, 0) x (1, 0, 0)
ref_plane "to_Bolt_1_205_YZ" through (285.6459, 0, -300) normal (1, 0, 0) x (0, 0, -1)
ref_plane "to_Bolt_1_205_ZX" through (285.6459, 0, -300) normal (0, 0, -1) x (0, 1, 0)
ref_plane "to_Bolt_1_206_XY" through (288.5167, 0, -300) normal (0, 1, 0) x (1, 0, 0)
ref_plane "to_Bolt_1_206_YZ" through (288.5167, 0, -300) normal (1, 0, 0) x (0, 0, -1)
ref_plane "to_Bolt_1_206_ZX" through (288.5167, 0, -300) normal (0, 0, -1) x (0, 1, 0)
ref_plane "to_Bolt_1_207_XY" through (291.3876, 0, -300) normal (0, 1, 0) x (1, 0, 0)
ref_plane "to_Bolt_1_207_YZ" through (291.3876, 0, -300) normal (1, 0, 0) x (0, 0, -1)
ref_plane "to_Bolt_1_207_ZX" through (291.3876, 0, -300) normal (0, 0, -1) x (0, 1, 0)
ref_plane "to_Bolt_1_208_XY" through (294.2584, 0, -300) normal (0, 1, 0) x (1, 0, 0)
ref_plane "to_Bolt_1_208_YZ" through (294.2584, 0, -300) normal (1, 0, 0) x (0, 0, -1)
ref_plane "to_Bolt_1_208_ZX" through (294.2584, 0, -300) normal (0, 0, -1) x (0, 1, 0)
ref_plane "to_Bolt_1_209_XY" through (297.1292, 0, -300) normal (0, 1, 0) x (1, 0, 0)
ref_plane "to_Bolt_1_209_YZ" through (297.1292, 0, -300) normal (1, 0, 0) x (0, 0, -1)
ref_plane "to_Bolt_1_209_ZX" through (297.1292, 0, -300) normal (0, 0, -1) x (0, 1, 0)
ref_plane "to_Bolt_1_21_XY" through (-242.5837, 0, -300) normal (0, 1, 0) x (1, 0, 0)
ref_plane "to_Bolt_1_21_YZ" through (-242.5837, 0, -300) normal (1, 0, 0) x (0, 0, -1)
ref_plane "to_Bolt_1_21_ZX" through (-242.5837, 0, -300) normal (0, 0, -1) x (0, 1, 0)
ref_plane "to_Bolt_1_210_XY" through (300, 0, -300) normal (0, 1, 0) x (1, 0, 0)
ref_plane "to_Bolt_1_210_YZ" through (300, 0, -300) normal (1, 0, 0) x (0, 0, -1)
ref_plane "to_Bolt_1_210_ZX" through (300, 0, -300) normal (0, 0, -1) x (0, 1, 0)
ref_plane "to_Bolt_1_211_XY" through (-300, 0, 300) normal (0, 1, 0) x (1, 0, 0)
ref_plane "to_Bolt_1_211_YZ" through (-300, 0, 300) normal (1, 0, 0) x (0, 0, -1)
ref_plane "to_Bolt_1_211_ZX" through (-300, 0, 300) normal (0, 0, -1) x (0, 1, 0)
ref_plane "to_Bolt_1_212_XY" through (-297.1292, 0, 300) normal (0, 1, 0) x (1, 0, 0)
ref_plane "to_Bolt_1_212_YZ" through (-297.1292, 0, 300) normal (1, 0, 0) x (0, 0, -1)
ref_plane "to_Bolt_1_212_ZX" through (-297.1292, 0, 300) normal (0, 0, -1) x (0, 1, 0)
ref_plane "to_Bolt_1_213_XY" through (-294.2584, 0, 300) normal (0, 1, 0) x (1, 0, 0)
ref_plane "to_Bolt_1_213_YZ" through (-294.2584, 0, 300) normal (1, 0, 0) x (0, 0, -1)
ref_plane "to_Bolt_1_213_ZX" through (-294.2584, 0, 300) normal (0, 0, -1) x (0, 1, 0)
ref_plane "to_Bolt_1_214_XY" through (-291.3876, 0, 300) normal (0, 1, 0) x (1, 0, 0)
ref_plane "to_Bolt_1_214_YZ" through (-291.3876, 0, 300) normal (1, 0, 0) x (0, 0, -1)
ref_plane "to_Bolt_1_214_ZX" through (-291.3876, 0, 300) normal (0, 0, -1) x (0, 1, 0)
ref_plane "to_Bolt_1_215_XY" through (-288.5167, 0, 300) normal (0, 1, 0) x (1, 0, 0)
ref_plane "to_Bolt_1_215_YZ" through (-288.5167, 0, 300) normal (1, 0, 0) x (0, 0, -1)
ref_plane "to_Bolt_1_215_ZX" through (-288.5167, 0, 300) normal (0, 0, -1) x (0, 1, 0)
ref_plane "to_Bolt_1_216_XY" through (-285.6459, 0, 300) normal (0, 1, 0) x (1, 0, 0)
ref_plane "to_Bolt_1_216_YZ" through (-285.6459, 0, 300) normal (1, 0, 0) x (0, 0, -1)
ref_plane "to_Bolt_1_216_ZX" through (-285.6459, 0, 300) normal (0, 0, -1) x (0, 1, 0)
ref_plane "to_Bolt_1_217_XY" through (-282.7751, 0, 300) normal (0, 1, 0) x (1, 0, 0)
ref_plane "to_Bolt_1_217_YZ" through (-282.7751, 0, 300) normal (1, 0, 0) x (0, 0, -1)
ref_plane "to_Bolt_1_217_ZX" through (-282.7751, 0, 300) normal (0, 0, -1) x (0, 1, 0)
ref_plane "to_Bolt_1_218_XY" through (-279.9043, 0, 300) normal (0, 1, 0) x (1, 0, 0)
ref_plane "to_Bolt_1_218_YZ" through (-279.9043, 0, 300) normal (1, 0, 0) x (0, 0, -1)
ref_plane "to_Bolt_1_218_ZX" through (-279.9043, 0, 300) normal (0, 0, -1) x (0, 1, 0)
ref_plane "to_Bolt_1_219_XY" through (-277.0335, 0, 300) normal (0, 1, 0) x (1, 0, 0)
ref_plane "to_Bolt_1_219_YZ" through (-277.0335, 0, 300) normal (1, 0, 0) x (0, 0, -1)
ref_plane "to_Bolt_1_219_ZX" through (-277.0335, 0, 300) normal (0, 0, -1) x (0, 1, 0)
ref_plane "to_Bolt_1_22_XY" through (-239.7129, 0, -300) normal (0, 1, 0) x (1, 0, 0)
ref_plane "to_Bolt_1_22_YZ" through (-239.7129, 0, -300) normal (1, 0, 0) x (0, 0, -1)
ref_plane "to_Bolt_1_22_ZX" through (-239.7129, 0, -300) normal (0, 0, -1) x (0, 1, 0)
ref_plane "to_Bolt_1_220_XY" through (-274.1627, 0, 300) normal (0, 1, 0) x (1, 0, 0)
ref_plane "to_Bolt_1_220_YZ" through (-274.1627, 0, 300) normal (1, 0, 0) x (0, 0, -1)
ref_plane "to_Bolt_1_220_ZX" through (-274.1627, 0, 300) normal (0, 0, -1) x (0, 1, 0)
ref_plane "to_Bolt_1_221_XY" through (-271.2919, 0, 300) normal (0, 1, 0) x (1, 0, 0)
ref_plane "to_Bolt_1_221_YZ" through (-271.2919, 0, 300) normal (1, 0, 0) x (0, 0, -1)
ref_plane "to_Bolt_1_221_ZX" through (-271.2919, 0, 300) normal (0, 0, -1) x (0, 1, 0)
ref_plane "to_Bolt_1_222_XY" through (-268.4211, 0, 300) normal (0, 1, 0) x (1, 0, 0)
ref_plane "to_Bolt_1_222_YZ" through (-268.4211, 0, 300) normal (1, 0, 0) x (0, 0, -1)
ref_plane "to_Bolt_1_222_ZX" through (-268.4211, 0, 300) normal (0, 0, -1) x (0, 1, 0)
ref_plane "to_Bolt_1_223_XY" through (-265.5502, 0, 300) normal (0, 1, 0) x (1, 0, 0)
ref_plane "to_Bolt_1_223_YZ" through (-265.5502, 0, 300) normal (1, 0, 0) x (0, 0, -1)
ref_plane "to_Bolt_1_223_ZX" through (-265.5502, 0, 300) normal (0, 0, -1) x (0, 1, 0)
ref_plane "to_Bolt_1_224_XY" through (-262.6794, 0, 300) normal (0, 1, 0) x (1, 0, 0)
ref_plane "to_Bolt_1_224_YZ" through (-262.6794, 0, 300) normal (1, 0, 0) x (0, 0, -1)
ref_plane "to_Bolt_1_224_ZX" through (-262.6794, 0, 300) normal (0, 0, -1) x (0, 1, 0)
ref_plane "to_Bolt_1_225_XY" through (-259.8086, 0, 300) normal (0, 1, 0) x (1, 0, 0)
ref_plane "to_Bolt_1_225_YZ" through (-259.8086, 0, 300) normal (1, 0, 0) x (0, 0, -1)
ref_plane "to_Bolt_1_225_ZX" through (-259.8086, 0, 300) normal (0, 0, -1) x (0, 1, 0)
ref_plane "to_Bolt_1_226_XY" through (-256.9378, 0, 300) normal (0, 1, 0) x (1, 0, 0)
ref_plane "to_Bolt_1_226_YZ" through (-256.9378, 0, 300) normal (1, 0, 0) x (0, 0, -1)
ref_plane "to_Bolt_1_226_ZX" through (-256.9378, 0, 300) normal (0, 0, -1) x (0, 1, 0)
ref_plane "to_Bolt_1_227_XY" through (-254.067, 0, 300) normal (0, 1, 0) x (1, 0, 0)
ref_plane "to_Bolt_1_227_YZ" through (-254.067, 0, 300) normal (1, 0, 0) x (0, 0, -1)
ref_plane "to_Bolt_1_227_ZX" through (-254.067, 0, 300) normal (0, 0, -1) x (0, 1, 0)
ref_plane "to_Bolt_1_228_XY" through (-251.1962, 0, 300) normal (0, 1, 0) x (1, 0, 0)
ref_plane "to_Bolt_1_228_YZ" through (-251.1962, 0, 300) normal (1, 0, 0) x (0, 0, -1)
ref_plane "to_Bolt_1_228_ZX" through (-251.1962, 0, 300) normal (0, 0, -1) x (0, 1, 0)
ref_plane "to_Bolt_1_229_XY" through (-248.3254, 0, 300) normal (0, 1, 0) x (1, 0, 0)
ref_plane "to_Bolt_1_229_YZ" through (-248.3254, 0, 300) normal (1, 0, 0) x (0, 0, -1)
ref_plane "to_Bolt_1_229_ZX" through (-248.3254, 0, 300) normal (0, 0, -1) x (0, 1, 0)
ref_plane "to_Bolt_1_23_XY" through (-236.8421, 0, -300) normal (0, 1, 0) x (1, 0, 0)
ref_plane "to_Bolt_1_23_YZ" through (-236.8421, 0, -300) normal (1, 0, 0) x (0, 0, -1)
ref_plane "to_Bolt_1_23_ZX" through (-236.8421, 0, -300) normal (0, 0, -1) x (0, 1, 0)
ref_plane "to_Bolt_1_230_XY" through (-245.4545, 0, 300) normal (0, 1, 0) x (1, 0, 0)
ref_plane "to_Bolt_1_230_YZ" through (-245.4545, 0, 300) normal (1, 0, 0) x (0, 0, -1)
ref_plane "to_Bolt_1_230_ZX" through (-245.4545, 0, 300) normal (0, 0, -1) x (0, 1, 0)
ref_plane "to_Bolt_1_231_XY" through (-242.5837, 0, 300) normal (0, 1, 0) x (1, 0, 0)
ref_plane "to_Bolt_1_231_YZ" through (-242.5837, 0, 300) normal (1, 0, 0) x (0, 0, -1)
ref_plane "to_Bolt_1_231_ZX" through (-242.5837, 0, 300) normal (0, 0, -1) x (0, 1, 0)
ref_plane "to_Bolt_1_232_XY" through (-239.7129, 0, 300) normal (0, 1, 0) x (1, 0, 0)
ref_plane "to_Bolt_1_232_YZ" through (-239.7129, 0, 300) normal (1, 0, 0) x (0, 0, -1)
ref_plane "to_Bolt_1_232_ZX" through (-239.7129, 0, 300) normal (0, 0, -1) x (0, 1, 0)
ref_plane "to_Bolt_1_233_XY" through (-236.8421, 0, 300) normal (0, 1, 0) x (1, 0, 0)
ref_plane "to_Bolt_1_233_YZ" through (-236.8421, 0, 300) normal (1, 0, 0) x (0, 0, -1)
ref_plane "to_Bolt_1_233_ZX" through (-236.8421, 0, 300) normal (0, 0, -1) x (0, 1, 0)
ref_plane "to_Bolt_1_234_XY" through (-233.9713, 0, 300) normal (0, 1, 0) x (1, 0, 0)
ref_plane "to_Bolt_1_234_YZ" through (-233.9713, 0, 300) normal (1, 0, 0) x (0, 0, -1)
ref_plane "to_Bolt_1_234_ZX" through (-233.9713, 0, 300) normal (0, 0, -1) x (0, 1, 0)
ref_plane "to_Bolt_1_235_XY" through (-231.1005, 0, 300) normal (0, 1, 0) x (1, 0, 0)
ref_plane "to_Bolt_1_235_YZ" through (-231.1005, 0, 300) normal (1, 0, 0) x (0, 0, -1)
ref_plane "to_Bolt_1_235_ZX" through (-231.1005, 0, 300) normal (0, 0, -1) x (0, 1, 0)
ref_plane "to_Bolt_1_236_XY" through (-228.2297, 0, 300) normal (0, 1, 0) x (1, 0, 0)
ref_plane "to_Bolt_1_236_YZ" through (-228.2297, 0, 300) normal (1, 0, 0) x (0, 0, -1)
ref_plane "to_Bolt_1_236_ZX" through (-228.2297, 0, 300) normal (0, 0, -1) x (0, 1, 0)
ref_plane "to_Bolt_1_237_XY" through (-225.3589, 0, 300) normal (0, 1, 0) x (1, 0, 0)
ref_plane "to_Bolt_1_237_YZ" through (-225.3589, 0, 300) normal (1, 0, 0) x (0, 0, -1)
ref_plane "to_Bolt_1_237_ZX" through (-225.3589, 0, 300) normal (0, 0, -1) x (0, 1, 0)
ref_plane "to_Bolt_1_238_XY" through (-222.488, 0, 300) normal (0, 1, 0) x (1, 0, 0)
ref_plane "to_Bolt_1_238_YZ" through (-222.488, 0, 300) normal (1, 0, 0) x (0, 0, -1)
ref_plane "to_Bolt_1_238_ZX" through (-222.488, 0, 300) normal (0, 0, -1) x (0, 1, 0)
ref_plane "to_Bolt_1_239_XY" through (-219.6172, 0, 300) normal (0, 1, 0) x (1, 0, 0)
ref_plane "to_Bolt_1_239_YZ" through (-219.6172, 0, 300) normal (1, 0, 0) x (0, 0, -1)
ref_plane "to_Bolt_1_239_ZX" through (-219.6172, 0, 300) normal (0, 0, -1) x (0, 1, 0)
ref_plane "to_Bolt_1_24_XY" through (-233.9713, 0, -300) normal (0, 1, 0) x (1, 0, 0)
ref_plane "to_Bolt_1_24_YZ" through (-233.9713, 0, -300) normal (1, 0, 0) x (0, 0, -1)
ref_plane "to_Bolt_1_24_ZX" through (-233.9713, 0, -300) normal (0, 0, -1) x (0, 1, 0)
ref_plane "to_Bolt_1_240_XY" through (-216.7464, 0, 300) normal (0, 1, 0) x (1, 0, 0)
ref_plane "to_Bolt_1_240_YZ" through (-216.7464, 0, 300) normal (1, 0, 0) x (0, 0, -1)
ref_plane "to_Bolt_1_240_ZX" through (-216.7464, 0, 300) normal (0, 0, -1) x (0, 1, 0)
ref_plane "to_Bolt_1_241_XY" through (-213.8756, 0, 300) normal (0, 1, 0) x (1, 0, 0)
ref_plane "to_Bolt_1_241_YZ" through (-213.8756, 0, 300) normal (1, 0, 0) x (0, 0, -1)
ref_plane "to_Bolt_1_241_ZX" through (-213.8756, 0, 300) normal (0, 0, -1) x (0, 1, 0)
ref_plane "to_Bolt_1_242_XY" through (-211.0048, 0, 300) normal (0, 1, 0) x (1, 0, 0)
ref_plane "to_Bolt_1_242_YZ" through (-211.0048, 0, 300) normal (1, 0, 0) x (0, 0, -1)
ref_plane "to_Bolt_1_242_ZX" through (-211.0048, 0, 300) normal (0, 0, -1) x (0, 1, 0)
ref_plane "to_Bolt_1_243_XY" through (-208.134, 0, 300) normal (0, 1, 0) x (1, 0, 0)
ref_plane "to_Bolt_1_243_YZ" through (-208.134, 0, 300) normal (1, 0, 0) x (0, 0, -1)
ref_plane "to_Bolt_1_243_ZX" through (-208.134, 0, 300) normal (0, 0, -1) x (0, 1, 0)
ref_plane "to_Bolt_1_244_XY" through (-205.2632, 0, 300) normal (0, 1, 0) x (1, 0, 0)
ref_plane "to_Bolt_1_244_YZ" through (-205.2632, 0, 300) normal (1, 0, 0) x (0, 0, -1)
ref_plane "to_Bolt_1_244_ZX" through (-205.2632, 0, 300) normal (0, 0, -1) x (0, 1, 0)
ref_plane "to_Bolt_1_245_XY" through (-202.3923, 0, 300) normal (0, 1, 0) x (1, 0, 0)
ref_plane "to_Bolt_1_245_YZ" through (-202.3923, 0, 300) normal (1, 0, 0) x (0, 0, -1)
ref_plane "to_Bolt_1_245_ZX" through (-202.3923, 0, 300) normal (0, 0, -1) x (0, 1, 0)
ref_plane "to_Bolt_1_246_XY" through (-199.5215, 0, 300) normal (0, 1, 0) x (1, 0, 0)
ref_plane "to_Bolt_1_246_YZ" through (-199.5215, 0, 300) normal (1, 0, 0) x (0, 0, -1)
ref_plane "to_Bolt_1_246_ZX" through (-199.5215, 0, 300) normal (0, 0, -1) x (0, 1, 0)
ref_plane "to_Bolt_1_247_XY" through (-196.6507, 0, 300) normal (0, 1, 0) x (1, 0, 0)
ref_plane "to_Bolt_1_247_YZ" through (-196.6507, 0, 300) normal (1, 0, 0) x (0, 0, -1)
ref_plane "to_Bolt_1_247_ZX" through (-196.6507, 0, 300) normal (0, 0, -1) x (0, 1, 0)
ref_plane "to_Bolt_1_248_XY" through (-193.7799, 0, 300) normal (0, 1, 0) x (1, 0, 0)
ref_plane "to_Bolt_1_248_YZ" through (-193.7799, 0, 300) normal (1, 0, 0) x (0, 0, -1)
ref_plane "to_Bolt_1_248_ZX" through (-193.7799, 0, 300) normal (0, 0, -1) x (0, 1, 0)
ref_plane "to_Bolt_1_249_XY" through (-190.9091, 0, 300) normal (0, 1, 0) x (1, 0, 0)
ref_plane "to_Bolt_1_249_YZ" through (-190.9091, 0, 300) normal (1, 0, 0) x (0, 0, -1)
ref_plane "to_Bolt_1_249_ZX" through (-190.9091, 0, 300) normal (0, 0, -1) x (0, 1, 0)
ref_plane "to_Bolt_1_25_XY" through (-231.1005, 0, -300) normal (0, 1, 0) x (1, 0, 0)
ref_plane "to_Bolt_1_25_YZ" through (-231.1005, 0, -300) normal (1, 0, 0) x (0, 0, -1)
ref_plane "to_Bolt_1_25_ZX" through (-231.1005, 0, -300) normal (0, 0, -1) x (0, 1, 0)
ref_plane "to_Bolt_1_250_XY" through (-188.0383, 0, 300) normal (0, 1, 0) x (1, 0, 0)
ref_plane "to_Bolt_1_250_YZ" through (-188.0383, 0, 300) normal (1, 0, 0) x (0, 0, -1)
ref_plane "to_Bolt_1_250_ZX" through (-188.0383, 0, 300) normal (0, 0, -1) x (0, 1, 0)
ref_plane "to_Bolt_1_251_XY" through (-185.1675, 0, 300) normal (0, 1, 0) x (1, 0, 0)
ref_plane "to_Bolt_1_251_YZ" through (-185.1675, 0, 300) normal (1, 0, 0) x (0, 0, -1)
ref_plane "to_Bolt_1_251_ZX" through (-185.1675, 0, 300) normal (0, 0, -1) x (0, 1, 0)
ref_plane "to_Bolt_1_252_XY" through (-182.2967, 0, 300) normal (0, 1, 0) x (1, 0, 0)
ref_plane "to_Bolt_1_252_YZ" through (-182.2967, 0, 300) normal (1, 0, 0) x (0, 0, -1)
ref_plane "to_Bolt_1_252_ZX" through (-182.2967, 0, 300) normal (0, 0, -1) x (0, 1, 0)
ref_plane "to_Bolt_1_253_XY" through (-179.4258, 0, 300) normal (0, 1, 0) x (1, 0, 0)
ref_plane "to_Bolt_1_253_YZ" through (-179.4258, 0, 300) normal (1, 0, 0) x (0, 0, -1)
ref_plane "to_Bolt_1_253_ZX" through (-179.4258, 0, 300) normal (0, 0, -1) x (0, 1, 0)
ref_plane "to_Bolt_1_254_XY" through (-176.555, 0, 300) normal (0, 1, 0) x (1, 0, 0)
ref_plane "to_Bolt_1_254_YZ" through (-176.555, 0, 300) normal (1, 0, 0) x (0, 0, -1)
ref_plane "to_Bolt_1_254_ZX" through (-176.555, 0, 300) normal (0, 0, -1) x (0, 1, 0)
ref_plane "to_Bolt_1_255_XY" through (-173.6842, 0, 300) normal (0, 1, 0) x (1, 0, 0)
ref_plane "to_Bolt_1_255_YZ" through (-173.6842, 0, 300) normal (1, 0, 0) x (0, 0, -1)
ref_plane "to_Bolt_1_255_ZX" through (-173.6842, 0, 300) normal (0, 0, -1) x (0, 1, 0)
ref_plane "to_Bolt_1_256_XY" through (-170.8134, 0, 300) normal (0, 1, 0) x (1, 0, 0)
ref_plane "to_Bolt_1_256_YZ" through (-170.8134, 0, 300) normal (1, 0, 0) x (0, 0, -1)
ref_plane "to_Bolt_1_256_ZX" through (-170.8134, 0, 300) normal (0, 0, -1) x (0, 1, 0)
ref_plane "to_Bolt_1_257_XY" through (-167.9426, 0, 300) normal (0, 1, 0) x (1, 0, 0)
ref_plane "to_Bolt_1_257_YZ" through (-167.9426, 0, 300) normal (1, 0, 0) x (0, 0, -1)
ref_plane "to_Bolt_1_257_ZX" through (-167.9426, 0, 300) normal (0, 0, -1) x (0, 1, 0)
ref_plane "to_Bolt_1_258_XY" through (-165.0718, 0, 300) normal (0, 1, 0) x (1, 0, 0)
ref_plane "to_Bolt_1_258_YZ" through (-165.0718, 0, 300) normal (1, 0, 0) x (0, 0, -1)
ref_plane "to_Bolt_1_258_ZX" through (-165.0718, 0, 300) normal (0, 0, -1) x (0, 1, 0)
ref_plane "to_Bolt_1_259_XY" through (-162.201, 0, 300) normal (0, 1, 0) x (1, 0, 0)
ref_plane "to_Bolt_1_259_YZ" through (-162.201, 0, 300) normal (1, 0, 0) x (0, 0, -1)
ref_plane "to_Bolt_1_259_ZX" through (-162.201, 0, 300) normal (0, 0, -1) x (0, 1, 0)
ref_plane "to_Bolt_1_26_XY" through (-228.2297, 0, -300) normal (0, 1, 0) x (1, 0, 0)